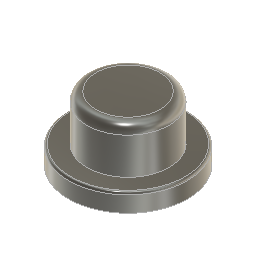
ShieldXL Batt Case Power Switch (Autodesk Fusion 360 design; units mm, degrees)
Autodesk Fusion 360 part; units mm, degrees
sketch "Sketch1" plane through (0, 0, 0) normal (0, 0, 1) x (1, 0, 0)
  circle A0 centre (0, 0) radius 3.25
  dimension "d1" = 6.5
  constraint coincident A0.centre origin
  measures "d1" diameter of A0
extrude "Extrude1" add sketch "Sketch1" along normal blind 1
sketch "Sketch2" plane through (0, 0, 1) normal (0, 0, 1) x (-1, 0, 0)
  circle A0 centre (0, 0) radius 3.25
  circle A1 centre (0, 0) radius 2.25
  dimension "d4" = 4.5
  constraint coincident A0.centre A1.centre
  measures "d4" diameter of A1
extrude "Extrude2" add sketch "Sketch2" along normal blind 2.5 contours A1
fillet "Fillet1" radius 0.5 1 edges at (2.0977, 0.8136, 3.5)
fillet "Fillet2" radius 0.125 1 edges at (-3.0301, -1.1753, 1)
sketch "Sketch3" plane through (0, 0, 0) normal (0, 0, 1) x (1, 0, 0)
  circle A0 centre (0, 0) radius 1.25
  dimension "d11" = 2.5
  constraint coincident A0.centre origin
  measures "d11" diameter of A0
extrude "Extrude3" cut sketch "Sketch3" along normal blind 0.5
